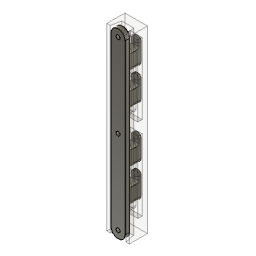
model (Autodesk Fusion 360 design; units mm, degrees)
Autodesk Fusion 360 part; units mm, degrees
sketch "Sketch1" plane through (0, 0, 0) normal (0, 1, 0) x (1, 0, 0)
  line L0 (0, 0) -> (25.4, 0)
  line L1 (25.4, 0) -> (25.4, -202.5)
  line L2 (25.4, -202.5) -> (0, -202.5)
  line L3 (0, -202.5) -> (0, 0)
  line L4 (6, -202.5) -> (6, 0)
  line L5 (19.4, 0) -> (19.4, -202.5)
  line L6 (8.1, -156.45) -> (8.1, -176.7)
  arc A0 (8.1, -176.7) -> (17.3, -176.7) centre (12.7, -176.7) ccw
  line L7 (17.3, -176.7) -> (17.3, -156.45)
  arc A1 (17.3, -156.45) -> (8.1, -156.45) centre (12.7, -156.45) ccw
  line L8 (6, -202.5) -> (12.7, -176.7) construction
  line L9 (12.7, -176.7) -> (19.4, -202.5) construction
  line L10 (0, -101.25) -> (25.4, -101.25) construction
  line L11 (8.1, -120) -> (8.1, -140.25)
  arc A2 (8.1, -140.25) -> (17.3, -140.25) centre (12.7, -140.25) ccw
  arc A3 (17.3, -120) -> (8.1, -120) centre (12.7, -120) ccw
  line L12 (17.3, -140.25) -> (17.3, -120)
  line L13 (8.1, -46.05) -> (8.1, -25.8)
  arc A4 (17.3, -25.8) -> (8.1, -25.8) centre (12.7, -25.8) ccw
  arc A5 (8.1, -46.05) -> (17.3, -46.05) centre (12.7, -46.05) ccw
  line L14 (17.3, -25.8) -> (17.3, -46.05)
  line L15 (8.1, -82.5) -> (8.1, -62.25)
  arc A6 (17.3, -62.25) -> (8.1, -62.25) centre (12.7, -62.25) ccw
  arc A7 (8.1, -82.5) -> (17.3, -82.5) centre (12.7, -82.5) ccw
  line L16 (17.3, -62.25) -> (17.3, -82.5)
  line L17 (6, -14.2) -> (19.4, -14.2)
  line L18 (6, -94.3) -> (19.4, -94.3)
  line L19 (6, -108.2) -> (19.4, -108.2)
  line L20 (6, -188.3) -> (19.4, -188.3)
  point P0 (12.7, -181.3)
  point P1 (12.7, -181.3)
  point P2 (12.7, -151.85)
  dimension "d1" = 202.5
  dimension "d2" = 25.4
  dimension "d3" = 6
  dimension "d4" = 6
  dimension "d5" = 9.2
  dimension "d7" = 21.2
  dimension "d8" = 29.45
  dimension "d11" = 0
  dimension "d12" = 36.45
  dimension "d17" = 14.2
  dimension "d18" = 6.95
  constraint horizontal L0
  constraint vertical L1
  constraint horizontal L2
  constraint vertical L3
  constraint coincident L0.start L3.end
  constraint coincident L2 L4.start
  constraint coincident L0 L4.end
  constraint coincident L0 L5.start
  constraint coincident L2 L5.end
  constraint vertical L5
  constraint vertical L4
  constraint tangent L6 A0
  constraint tangent L6 A1
  constraint tangent L7 A1
  constraint tangent A0 L7
  constraint vertical L6
  constraint vertical L7
  constraint coincident A0.centre L8.end
  constraint equal L8 L9
  constraint midpoint L3 L10.start
  constraint midpoint L1 L10.end
  constraint midpoint A0 P1
  constraint midpoint A1 P2
  constraint symmetric L6.start L10 L13.start
  constraint symmetric L6.end L10 L13.end
  constraint symmetric A0.end L10 A4.start
  constraint symmetric A0 L10 A4
  constraint symmetric L7.end L10 A5.end
  constraint symmetric A1 L10 A5
  constraint symmetric L10 L11.start L15.start
  constraint symmetric L10 L11.end L15.end
  constraint symmetric L10 A2.end A6.start
  constraint symmetric L10 A2 A6
  constraint symmetric L10 A3.start A7.end
  constraint symmetric L10 A3 A7
  constraint coincident L4 L17.start
  constraint coincident L5 L17.end
  constraint horizontal L17
  constraint coincident L4 L18.start
  constraint coincident L5 L18.end
  constraint horizontal L18
  constraint symmetric L10 L17.start L20.start
  constraint symmetric L10 L17.end L20.end
  constraint symmetric L10 L18.start L19.start
  constraint symmetric L10 L18.end L19.end
  measures "d1" distance of L0.start L2.end
  measures "d2" distance of L1.end L2.end
  measures "d3" distance of L2.end L4.start
  measures "d4" distance of L1.end L5.end
  measures "d5" distance of L6.end A0.end
  measures "d7" distance of L2 P1
  measures "d8" distance of P1 P2
  measures "d17" vertical distance of L0.start L17.start
  measures "d18" vertical distance of L10.start L18.start
extrude "Extrude1" add sketch "Sketch1" against normal blind 20.4 contours L0 L2 L3 L4 | L0 L1 L2 L5 makes body 1 at (6, -6.8, 135) makes body 2 at (25.4, -6.8, 67.5)
extrude "Extrude2" add sketch "Sketch1" against normal blind 9.55 contours L0 L4 L5 L17 | L4 L5 L17 L18 | L2 L4 L5 L20 | L4 L5 L18 L19 | L4 L5 L19 L20 bodies 1 2
extrude "Extrude3" cut sketch "Sketch1" against normal blind 4.8 contours L4 L5 L17 L18 | L4 L5 L19 L20 bodies 1
draft "Draft1" angle 11 neutral plane through (0, -9.55, 0) pull (0, -1, 0) 2 faces at (6, -13.1667, 135) (19.4, -13.1667, 67.5) on bodies 1
sketch "Sketch2" plane through (0, -9.55, 0) normal (0, -1, 0) x (1, 0, 0)
  line L0 (17.3, 140.25) -> (17.3, 120)
  arc A0 (8.1, 120) -> (17.3, 120) centre (12.7, 120) ccw
  line L1 (8.1, 120) -> (8.1, 140.25)
  arc A1 (17.3, 140.25) -> (8.1, 140.25) centre (12.7, 140.25) ccw
  arc A2 (17.3, 82.5) -> (8.1, 82.5) centre (12.7, 82.5) ccw
  line L2 (17.3, 82.5) -> (17.3, 62.25)
  arc A3 (8.1, 62.25) -> (17.3, 62.25) centre (12.7, 62.25) ccw
  line L3 (8.1, 62.25) -> (8.1, 82.5)
  arc A4 (17.3, 46.05) -> (8.1, 46.05) centre (12.7, 46.05) ccw
  line L4 (17.3, 46.05) -> (17.3, 25.8)
  arc A5 (8.1, 25.8) -> (17.3, 25.8) centre (12.7, 25.8) ccw
  line L5 (8.1, 25.8) -> (8.1, 46.05)
  arc A6 (8.1, 156.45) -> (17.3, 156.45) centre (12.7, 156.45) ccw
  line L6 (8.1, 156.45) -> (8.1, 176.7)
  arc A7 (17.3, 176.7) -> (8.1, 176.7) centre (12.7, 176.7) ccw
  line L7 (17.3, 176.7) -> (17.3, 156.45)
  line L8 (6, 0) -> (19.4, 0)
  line L9 (19.4, 0) -> (19.4, 202.5)
  line L10 (19.4, 202.5) -> (6, 202.5)
  line L11 (6, 202.5) -> (6, 0)
  line L12 (19.4, 188.3) -> (6, 188.3)
  line L13 (6, 108.2) -> (19.4, 108.2)
  line L14 (19.4, 94.3) -> (6, 94.3)
  line L15 (6, 14.2) -> (19.4, 14.2)
  line L16 (8.35, 156.45) -> (8.35, 176.7)
  arc A8 (17.05, 176.7) -> (8.35, 176.7) centre (12.7, 176.7) ccw
  line L17 (17.05, 176.7) -> (17.05, 156.45)
  arc A9 (8.35, 156.45) -> (17.05, 156.45) centre (12.7, 156.45) ccw
  line L18 (8.35, 162.45) -> (8.35, 182.7)
  arc A10 (8.35, 162.45) -> (17.05, 162.45) centre (12.7, 162.45) ccw
  line L19 (17.05, 182.7) -> (17.05, 162.45)
  arc A11 (17.05, 182.7) -> (8.35, 182.7) centre (12.7, 182.7) ccw
  arc A12 (8.35, 120) -> (17.05, 120) centre (12.7, 120) ccw
  line L20 (17.05, 140.25) -> (17.05, 120)
  arc A13 (17.05, 140.25) -> (8.35, 140.25) centre (12.7, 140.25) ccw
  line L21 (8.35, 120) -> (8.35, 140.25)
  line L22 (8.35, 62.25) -> (8.35, 82.5)
  arc A14 (17.05, 82.5) -> (8.35, 82.5) centre (12.7, 82.5) ccw
  line L23 (17.05, 82.5) -> (17.05, 62.25)
  arc A15 (8.35, 62.25) -> (17.05, 62.25) centre (12.7, 62.25) ccw
  line L24 (8.35, 25.8) -> (8.35, 46.05)
  arc A16 (17.05, 46.05) -> (8.35, 46.05) centre (12.7, 46.05) ccw
  line L25 (17.05, 46.05) -> (17.05, 25.8)
  arc A17 (8.35, 25.8) -> (17.05, 25.8) centre (12.7, 25.8) ccw
  line L26 (8.35, 126) -> (8.35, 146.25)
  arc A18 (8.35, 126) -> (17.05, 126) centre (12.7, 126) ccw
  line L27 (17.05, 146.25) -> (17.05, 126)
  arc A19 (17.05, 146.25) -> (8.35, 146.25) centre (12.7, 146.25) ccw
  line L28 (8.35, 68.25) -> (8.35, 88.5)
  arc A20 (8.35, 68.25) -> (17.05, 68.25) centre (12.7, 68.25) ccw
  line L29 (17.05, 88.5) -> (17.05, 68.25)
  arc A21 (17.05, 88.5) -> (8.35, 88.5) centre (12.7, 88.5) ccw
  line L30 (8.35, 31.8) -> (8.35, 52.05)
  arc A22 (8.35, 31.8) -> (17.05, 31.8) centre (12.7, 31.8) ccw
  line L31 (17.05, 52.05) -> (17.05, 31.8)
  arc A23 (17.05, 52.05) -> (8.35, 52.05) centre (12.7, 52.05) ccw
  line L32 (12.7, 202.5) -> (12.7, 0) construction
  circle A24 centre (12.7, 195.4) radius 2.25
  circle A25 centre (12.7, 101.25) radius 2.25
  circle A26 centre (12.7, 7.1) radius 2.25
  line L33 (6, 188.3) -> (12.7, 195.4) construction
  line L34 (6, 202.5) -> (12.7, 195.4) construction
  line L35 (6, 14.2) -> (12.7, 7.1) construction
  line L36 (6, 0) -> (12.7, 7.1) construction
  line L37 (19.15, 0.25) -> (19.15, 202.25)
  line L38 (19.15, 202.25) -> (6.25, 202.25)
  line L39 (6.25, 202.25) -> (6.25, 0.25)
  line L40 (6.25, 0.25) -> (19.15, 0.25)
  dimension "d21" = -0.25
  dimension "d24" = 0
  dimension "d25" = 6
  dimension "d26" = 0.25
  dimension "d27" = -0.25
  dimension "d28" = -0.25
  dimension "d29" = 4.5
  dimension "d30" = -0.25
  constraint midpoint L10 L32.start
  constraint midpoint L8 L32.end
  constraint coincident L32 A24.centre
  constraint midpoint L32 A25.centre
  constraint equal A24 A25
  constraint coincident L32 A26.centre
  constraint equal A25 A26
  constraint coincident L12.end L33.start
  constraint coincident A24.centre L33.end
  constraint coincident L10.end L11.start
  constraint coincident L15.start L35.start
  constraint coincident A26.centre L35.end
  constraint coincident L8.start L11.end
  constraint equal L35 L36
  constraint equal L33 L34
  measures "d29" diameter of A24
extrude "Extrude4" add sketch "Sketch2" against normal blind 6 from surface at 10.85 separate body contours L0 A0 L1 A1 A12 L20 L21 L26 L27 | A1 A13 L26 L27 | A1 L26 L27 A19 | L20 A13 L21 L26 A18 L27 | A12 L20 L21 A18 | A2 L2 A3 L3 L22 L23 A15 L28 L29 | A2 A14 L28 L29 | A2 L28 L29 A21 | L22 A14 L23 L28 A20 L29 | L22 L23 A15 A20 | A4 L4 A5 L5 L24 L25 A17 L30 L31 | A4 A16 L30 L31 | A4 L30 L31 A23 | L24 A16 L25 L30 A22 L31 | L24 L25 A17 A22 | A6 L6 A7 L7 L16 L17 A9 L18 L19 | A7 L18 L19 A11 | A7 A8 L18 L19 | L16 A8 L17 L18 A10 L19 | L16 L17 A9 A10 | L14 L15 L37 L39 | L15 L37 L39 L40 | L13 L14 L37 L39 | L12 L13 L37 L39 | L12 L37 L38 L39 makes body 3
extrude "Extrude5" add sketch "Sketch2" along normal up to surface (4.85 mm away) and the other way up to surface (5.5 mm away) contours L20 A13 L21 L26 A18 L27 | L22 A14 L23 L28 A20 L29 | L24 A16 L25 L30 A22 L31 | L16 A8 L17 L18 A10 L19 bodies 3
extrude "Extrude6" add sketch "Sketch2" against normal blind 6 from surface at -5.5 contours A1 A13 L26 L27 | A1 L26 L27 A19 | L20 A13 L21 L26 A18 L27 | A2 A14 L28 L29 | A2 L28 L29 A21 | L22 A14 L23 L28 A20 L29 | A4 A16 L30 L31 | A4 L30 L31 A23 | L24 A16 L25 L30 A22 L31 | A7 L18 L19 A11 | A7 A8 L18 L19 | L16 A8 L17 L18 A10 L19 bodies 3
chamfer "Chamfer1" distance 3 angle 45 3 edges at (10.6023, -14.4, 194.5864) (10.6023, -14.4, 100.4364) (10.6023, -14.4, 6.2864) on bodies 3
fillet "Fillet1" radius 6.45 4 edges at (19.15, -17.4, 202.25) (6.25, -17.4, 202.25) (19.15, -17.4, 0.25) (6.25, -17.4, 0.25) on bodies 3
chamfer "Chamfer2" distance 3 angle 45 12 edges at (12.7, -4.05, 187.05) (8.35, -4.05, 179.7) (17.05, -4.05, 179.7) (12.7, -4.05, 150.6) (8.35, -4.05, 143.25) (17.05, -4.05, 143.25) (12.7, -4.05, 92.85) (8.35, -4.05, 85.5) (17.05, -4.05, 85.5) (12.7, -4.05, 56.4) (8.35, -4.05, 49.05) (17.05, -4.05, 49.05) on bodies 3
chamfer "Chamfer3" distance 1 angle 45 12 edges at (12.7, -4.05, 184.05) (14.05, -4.05, 181.7676) (11.35, -4.05, 181.7676) (12.7, -4.05, 147.6) (14.05, -4.05, 145.3176) (11.35, -4.05, 145.3176) (12.7, -4.05, 89.85) (14.05, -4.05, 87.5676) (11.35, -4.05, 87.5676) (14.05, -4.05, 51.1176) (11.35, -4.05, 51.1176) (12.7, -4.05, 53.4) on bodies 3
move_face "OffsetFaces1" offset 1.5 2 faces at (19.15, -16.4, 69.7329) (6.25, -16.4, 69.7329) on bodies 3
fillet "Fillet2" radius 3 16 edges at (8.35, -14.4, 169.575) (12.7, -14.4, 158.1) (17.05, -14.4, 169.575) (12.7, -14.4, 181.05) (8.35, -14.4, 133.125) (12.7, -14.4, 121.65) (17.05, -14.4, 133.125) (12.7, -14.4, 144.6) (8.35, -14.4, 75.375) (12.7, -14.4, 63.9) (17.05, -14.4, 75.375) (12.7, -14.4, 86.85) (12.7, -14.4, 27.45) (17.05, -14.4, 38.925) (12.7, -14.4, 50.4) (8.35, -14.4, 38.925) on bodies 3
chamfer "Chamfer4" distance 1 angle 45 4 edges at (20.65, -14.4, 101.25) (12.7, -14.4, -1.25) (4.75, -14.4, 101.25) (12.7, -14.4, 203.75) 4 faces at (11.25, 1.95, 45.3) (14.15, 1.95, 81.75) (14.15, 1.95, 132.75) (11.25, 1.95, 169.2) on bodies 3
equation "d2 = 1\""
equation "d4 = d3"
equation "d12 = d8 + 7 mm"
equation "d18 = ( 13.9 / 2 ) * 1 mm"
